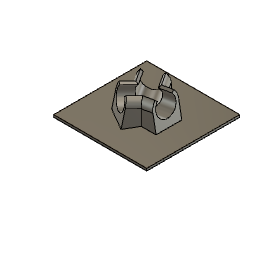
3servojoint v3 (Autodesk Fusion 360 design; units mm, degrees)
Autodesk Fusion 360 part; units mm, degrees
sketch "スケッチ1" plane through (0, 0, 0) normal (0, 1, 0) x (1, 0, 0)
  line L0 (15, -15) -> (-15, -15)
  line L1 (-15, -15) -> (-15, 15)
  line L2 (-15, 15) -> (15, 15)
  line L3 (15, 15) -> (15, -15)
  line L4 (15, -15) -> (-15, 15) construction
  line L5 (-15, -15) -> (15, 15) construction
  dimension "d1" = 30
  dimension "d2" = 30
  constraint perpendicular L0 L1
  constraint parallel L0 L2
  constraint parallel L1 L3
  constraint horizontal L0
  constraint coincident L4 origin
  constraint coincident L5 origin
  measures "d1" distance of L1.end L2.end
  measures "d2" distance of L0.end L1.end
sketch "スケッチ2" plane through (0, 0, 0) normal (1, 0, 0) x (0, 0, -1)
extrude "押し出し1" add sketch "スケッチ1" along normal blind 0.75 makes body 1
sketch "スケッチ3" plane through (0, 0.75, 0) normal (0, 1, 0) x (-1, 0, 0)
  line L0 (-15, -15) -> (15, -15)
  line L1 (15, -15) -> (15, 15)
  line L2 (15, 15) -> (-15, 15)
  line L3 (-15, 15) -> (-15, -15)
sketch "スケッチ4" plane through (0, 0, 0) normal (1, 0, 0) x (0, 0, -1)
  line L0 (0, 0.75) -> (0, 9.05)
  circle A0 centre (0, 4.9) radius 4.15
  circle A1 centre (0, 4.9) radius 3.25
  line L1 (0, 0.75) -> (-4.15, 0.75)
  line L2 (-4.15, 0.75) -> (-4.15, 4.9)
  line L3 (0, 0.75) -> (4.15, 0.75)
  line L4 (4.15, 0.75) -> (4.15, 4.9)
  line L5 (0, 4.9) -> (3.173, 7.5625)
  line L6 (0, 4.9) -> (4.15, 4.9) construction
  line L7 (0, 4.9) -> (-3.173, 7.5625)
  line L8 (0, 4.9) -> (4.15, 4.9) construction
  point P0 (0, 0.75)
  dimension "d5" = 8.3
  dimension "d6" = 6.5
  dimension "d7" = 4.15
  dimension "d16" = 40
  dimension "d17" = 140
  constraint coincident P0 L0.start
  constraint vertical L0
  constraint midpoint L0 A0.centre
  constraint coincident L0.end A0
  constraint concentric A0 A1
  constraint perpendicular L0 L1
  constraint coincident A0 L2.end
  constraint tangent A0 L2
  constraint symmetric P0 L0 L1.start
  constraint symmetric L0 L1.end L3.end
  constraint symmetric L0 L2.end L4.end
  constraint horizontal L6
  constraint coincident A0.centre A1.centre
  constraint horizontal L8
  measures "d5" distance of P0 L0.end
  measures "d6" diameter of A1
  measures "d7" distance of P0 L1.end
  measures "d16" angle of L5 L6
  measures "d17" angle of L7 L8
extrude "押し出し2" add sketch "スケッチ4" along normal blind 10 separate body contours L0 A0 A1 | A0 L1 L2 | L0 A0 A1 | A0 L3 L4 makes body 2
pattern_circular "C パターン1" count 3 over 360 about axis through (0, 1.75, 0) along (0, 1, 0) of bodies 2 makes body 3 at (-2.4189, 1.8263, -6.3014) makes body 4 at (-4.3725, 1.8796, 5.1735)
ref_plane "作業平面1" through (-2.5, 2.825, 4.3301) normal (0.866025, 0, 0.5) x (0, 1, 0)
sketch "スケッチ5" plane through (-2, 2.375, 3.4641) normal (0.866025, 0, 0.5) x (0, 1, 0)
ref_plane "作業平面2" through (-2.5, 2.825, -4.3301) normal (0.866025, 0, -0.5) x (0, -1, 0)
ref_plane "作業平面3" through (-2.5, 2.825, 4.3301) normal (0.866025, 0, 0.5) x (0, 1, 0)
split "分割1" by plane through (-2.5, 2.825, -4.3301) normal (0.866025, 0, -0.5) bodies 2 makes body 5 at (6.6667, 9.0453, -0.1975)
split "分割2" by plane through (-2.5, 2.825, 4.3301) normal (0.866025, 0, 0.5) bodies 5 makes body 6 at (6.7284, 1.6604, 0.2604)
pattern_circular "C パターン2" count 3 over 360 about axis through (0, 1.75, 0) along (0, 1, 0) of bodies 6 makes body 7 at (-3.1459, 1.6595, -5.9447) makes body 8 at (-3.5753, 1.6595, 5.6968)
ref_plane "作業平面4" through (0, 0, 12.125) normal (-0.984808, -0.173648, 0) x (0, 0, 1)
sketch "スケッチ6" plane through (0, 0, 12.125) normal (-0.984808, -0.173648, 0) x (0, 0, 1)
  circle A0 through (-8.875, 5.1348, -0.1736) (-13.75, 7.9494, -0.1736) (-13.75, 2.3202, -0.1736)
  circle A1 through (-7.975, 5.1348, -0.1736) (-14.2, 8.7288, -0.1736) (-14.2, 1.5408, -0.1736)
  line L0 (-12.125, 0.9848, -0.1736) -> (-12.125, 9.2848, -0.1736)
  line L1 (-7.975, 0.9848, -0.1736) -> (-7.975, 5.1348, -0.1736)
  line L2 (-12.125, 0.9848, -0.1736) -> (-7.975, 0.9848, -0.1736)
  line L3 (-12.125, 0.9848, -0.1736) -> (-16.275, 0.9848, -0.1736)
  line L4 (-16.275, 0.9848, -0.1736) -> (-16.275, 5.1348, -0.1736)
  line L5 (-12.125, 5.1348, -0.1736) -> (-15.1474, 7.9787, -0.1736)
  line L6 (-12.125, 5.1348, -0.1736) -> (-15.1474, 7.9787, -0.1736)
  line L7 (-12.125, 5.1348, -0.1736) -> (-9.1026, 7.9787, -0.1736)
ref_plane "作業平面5" through (0.171, 0.0302, 12.125) normal (-0.984808, -0.173648, 0) x (0, 0, 1)
extrude "押し出し3" add sketch "スケッチ6" against normal blind 7 separate body contours A0 A1 L0 L7 | A0 A1 L0 L5 L6 | A1 L3 L4 | A1 L1 L2 in plane through (0.171, 0.0301, 12.125) normal (-0.984808, -0.173648, 0) picked at (-0.0662, 1.3753, 0.7408) picked at (-0.6645, 4.7683, -3.8285) makes body 9
extrude "押し出し4" add 2 faces at (4.5957, 1.8103, -2.7667) (4.5957, 1.8103, 2.7667) along direction (0.173648, -0.984808, 0) blind 7 separate body on bodies 9 makes body 10
split "分割3" by plane through (0, 0.75, 0) normal (0, 1, 0) bodies 10 makes body 11 at (4.5957, 1.8103, 1.3833)
split "分割4" by plane through (0, 0, 0) normal (1, 0, 0) bodies 9 makes body 12 at (4.4827, 2.7912, -0.7408)
combine "結合1" operation add target body 12 tool bodies 11
split "分割5" by plane through (-2.5, 2.825, 4.3301) normal (0.866025, 0, 0.5) bodies 12 makes body 13 at (4.4828, 2.7932, 0.7492)
split "分割6" by plane through (-2.5, 2.825, -4.3301) normal (0.866025, 0, -0.5) bodies 13 makes body 14 at (4.5378, 2.723, 0.2392)
pattern_circular "C パターン3" count 3 over 360 about axis through (0, 1.75, 0) along (0, 1, 0) of bodies 14 makes body 15 at (-2.0595, 2.7237, -4.0533) makes body 16 at (-2.4805, 2.7237, 3.8103)
hidden bodies 2 3 4 5 6 7 8 9 10 12 13
